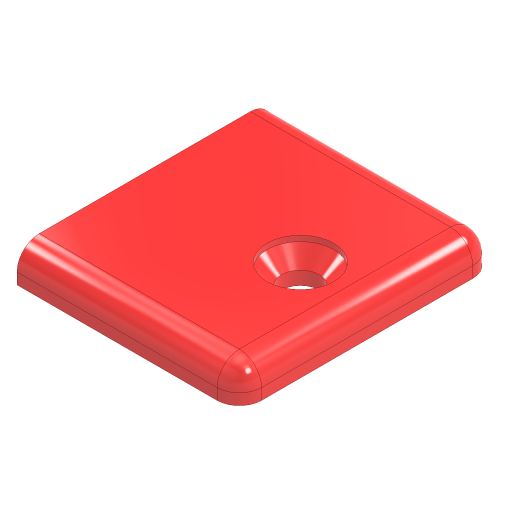
# Autodesk Inventor part: LIKA LKM-1439
Saved by Autodesk Inventor 2024.3 (Build 283343000, 343)
## iProperties
Created: 2025-06-09
Part Number: LIKA LKM-1439
Material: Generic
Document SubType Name: Modeling
Designer: MPA
Density: 1 g/cm^3
Appearance: Light Red
Author: MPA
Autodesk Inventor part; units mm, degrees
ref_plane "YZ Plane" through (0, 0, 0) normal (1, 0, 0) x (0, 1, 0)
ref_plane "XZ Plane" through (0, 0, 0) normal (0, 1, 0) x (-1, 0, 0)
ref_plane "XY Plane" through (0, 0, 0) normal (0, 0, 1) x (1, 0, 0)
sketch "Sketch1" plane through (0, 0, 0) normal (0, 1, 0) x (-1, 0, 0)
  line L0 (-10, 11.5) -> (10, 11.5)
  line L1 (10, 11.5) -> (10, -11.5)
  line L2 (10, -11.5) -> (-10, -11.5)
  line L3 (-10, -11.5) -> (-10, 11.5)
  line L4 (-10, 11.5) -> (10, -11.5) construction
  line L5 (10, 11.5) -> (-10, -11.5) construction
  point P0 (0, 0)
  dimension "d0" = 20
  dimension "d1" = 23
  constraints: 12 end point, 2 midpoint, 2 parallel, 1 horizontal, 1 perpendicular
  measures "d0" distance of L1.end L2.end
  measures "d1" distance of L0.end L1.end
extrude "Extrusion1" add sketch "Sketch1" along normal blind 3
sketch "Sketch2" plane through (0, 0, 0) normal (0, -1, 0) x (1, 0, 0)
  line L0 (10, -11.5) -> (-10, -11.5) projected
  line L1 (10, 11.5) -> (10, -11.5) projected
  line L2 (-10, 11.5) -> (10, 11.5) projected
  line L3 (-10, -11.5) -> (-10, 11.5) projected
  line L4 (0, -10.1) -> (-10, -10.1)
  line L5 (-10, -10.1) -> (-10, 10.1)
  line L6 (-10, 10.1) -> (0, 10.1)
  line L7 (0, 10.1) -> (0, -10.1)
  line L8 (0, -10.1) -> (-10, 10.1) construction
  line L9 (-10, -10.1) -> (0, 10.1) construction
  line L10 (-10, -11.5) -> (-10, 11.5) projected
  point P0 (0, 0)
  point P1 (-5, 0)
  dimension "d4" = 20.2
  dimension "d5" = 10
  constraints: 12 end point, 2 midpoint, 2 parallel, 1 horizontal, 1 horizontal alignment, 1 perpendicular, 1 point on line
  measures "d4" distance of L4.end L5.end
  measures "d5" distance of L5.end L6.end
extrude "Extrusion2" cut sketch "Sketch2" against normal blind 1.4 contours L3 L6 L7 L4
sketch "Sketch3" plane through (0, 3, 0) normal (0, 1, 0) x (1, 0, 0)
  line L0 (10, -11.5) -> (10, 11.5) projected
  point P0 (0, 0)
  point P1 (4, 0)
  dimension "d8" = 6
  constraints: 1 horizontal alignment
  measures "d8" distance from line of L0 point (4, 0)
hole "Hole1" at (4, 3, 0) direction (0, -1, 0) diameter 3.4 end through all counterbore diameter 6 counterbore depth 0.5
chamfer "Chamfer1" distance 1.3 angle 45 1 edges at (4, 2.5, -1.7)
fillet "Fillet1" radius 2 3 edges at (0, 3, 11.5) (10, 3, 0) (0, 3, -11.5)
fillet "Fillet2" radius 2 4 edges at (9.4142, 2.4142, 10.9142) (10, 0.5, 11.5) (9.4142, 2.4142, -10.9142) (10, 0.5, -11.5)
body "Solid1"
